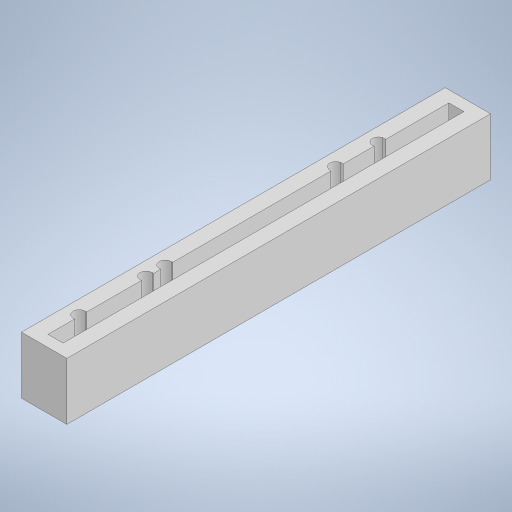
# Autodesk Inventor part: Microbit Breakout
Saved by Autodesk Inventor 2024.1 (Build 281209000, 209)
## iProperties
Created: 2023-12-30
Part Number: Microbit Breakout
Material: Generic
Document SubType Name: Modeling
Designer: ryanm
Density: 1 g/cm^3
Appearance: Default
Author: ryanm
Autodesk Inventor part; units mm, degrees
ref_plane "YZ Plane" through (0, 0, 0) normal (1, 0, 0) x (0, 1, 0)
ref_plane "XZ Plane" through (0, 0, 0) normal (0, 1, 0) x (-1, 0, 0)
ref_plane "XY Plane" through (0, 0, 0) normal (0, 0, 1) x (1, 0, 0)
sketch "Sketch1" plane through (0, 0, 0) normal (0, 1, 0) x (-1, 0, 0)
  line L0 (3, -28) -> (-3, -28)
  line L1 (-3, -28) -> (-3, 28)
  line L2 (-3, 28) -> (3, 28)
  line L3 (3, 28) -> (3, -28)
  point P0 (0, 0)
  point P1 (0, -28)
  point P2 (3, 0)
  dimension "d0" = 56
  dimension "d1" = 6
  constraints: 8 end point, 2 midpoint, 2 parallel, 1 horizontal, 1 horizontal alignment, 1 perpendicular, 1 vertical alignment
  measures "d0" distance of L2.end L0.start
  measures "d1" distance of L0.start L0.end
extrude "Extrusion1" add sketch "Sketch1" along normal blind 2
sketch "Sketch6" plane through (0, 2, 0) normal (0, 1, 0) x (1, 0, 0)
  line L0 (-3, 28) -> (-3, -28) projected
  line L1 (3, -28) -> (3, 28) projected
  line L2 (-3, 28) -> (3, 28)
  line L3 (3, 28) -> (3, -28)
  line L4 (3, -28) -> (-3, -28)
  line L5 (-3, -28) -> (-3, 28)
  point P0 (0, 0)
  constraints: 8 end point, 2 parallel, 1 horizontal, 1 perpendicular
extrude "Extrusion6" add sketch "Sketch6" along normal blind 5.56
sketch "Sketch4" plane through (0, 2, 0) normal (0, 1, 0) x (1, 0, 0)
  line L0 (-1, 26.5) -> (1, 26.5)
  line L1 (1, 26.5) -> (1, -26.5)
  line L2 (1, -26.5) -> (-1, -26.5)
  line L3 (-1, -26.5) -> (-1, 26.5)
  point P0 (0, 0)
  point P1 (0, 26.5)
  point P2 (-1, 0)
  dimension "d10" = 2
  dimension "d11" = 53
  constraints: 8 end point, 2 midpoint, 2 parallel, 1 horizontal, 1 horizontal alignment, 1 perpendicular, 1 vertical alignment
  measures "d10" distance of L0.start L0.end
  measures "d11" distance of L0.end L1.end
extrude "Extrusion4" cut sketch "Sketch4" along normal through all
sketch "Sketch5" plane through (0, 7.56, 0) normal (0, 1, 0) x (1, 0, 0)
  arc A0 (-1.4, 18.1546) -> (-1.4, 16.6054) centre (-1.2, 17.38) ccw
  line L0 (-1, 26.5) -> (-1, -26.5) projected
  line L1 (1, 26.5) -> (-1, 26.5) projected
  arc A1 (-1.4, 12.5246) -> (-1.3887, 10.9726) centre (-1.2, 11.75) ccw
  arc A2 (-1.2, -21.37) -> (-1.2, -22.97) centre (-1.2, -22.17) ccw
  arc A3 (-1.2, -12.54) -> (-1.2, -14.14) centre (-1.2, -13.34) ccw
  arc A4 (-1.2, -10) -> (-1.2, -11.6) centre (-1.2, -10.8) ccw
  line L2 (-1, -26.5) -> (1, -26.5) projected
  line L3 (-1.4, 18.1546) -> (-1, 18.1546)
  line L4 (-1.4, 16.6054) -> (-1, 16.6054)
  line L5 (-1.4, 12.5246) -> (-1, 12.5246)
  line L6 (-1.3887, 10.9726) -> (-1, 10.8782)
  line L7 (-1.2, -10) -> (-1, -10)
  line L8 (-1.2, -11.6) -> (-1, -11.6)
  line L9 (-1.2, -12.54) -> (-1, -12.54)
  line L10 (-1.2, -14.14) -> (-1, -14.14)
  line L11 (-1.2, -21.37) -> (-1, -21.37)
  line L12 (-1.2, -22.97) -> (-1, -22.97)
  point P0 (0, 0)
  dimension "d14" = 1.6
  dimension "d15" = 0.2
  dimension "d16" = 9.12
  dimension "d17" = 1.6
  dimension "d18" = 14.75
  dimension "d19" = 1.6
  dimension "d20" = 1.6
  dimension "d21" = 1.6
  dimension "d22" = 4.33
  dimension "d23" = 13.16
  dimension "d24" = 15.7
  dimension "d29" = 0.4
  dimension "d30" = 0.4
  dimension "d31" = 0.4
  dimension "d32" = 0.4
  constraints: 20 end point, 10 point on circle, 7 horizontal, 7 tangent, 5 centre point, 4 vertical alignment, 2 parallel, 11 other
  measures "d14" diameter of A0
  measures "d16" distance from line of A0.centre L1
  measures "d17" diameter of A1
  measures "d18" distance from line of A1.centre L1
  measures "d19" diameter of A2
  measures "d20" diameter of A3
  measures "d21" diameter of A4
  measures "d22" distance from line of L2 A2.centre
  measures "d23" distance from line of L2 A3.centre
  measures "d24" distance from line of L2 A4.centre
  measures "d29" distance of L4.start L4.end
  measures "d30" distance of L3.start L3.end
  measures "d31" distance of L6.start L6.end
  measures "d32" distance of L5.start L5.end
extrude "Extrusion5" cut sketch "Sketch5" against normal through all
equation "\"d30\" = d29"
body "Solid1"
